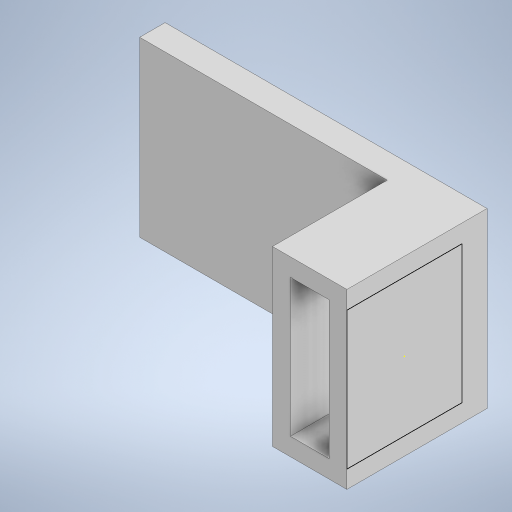
# Autodesk Inventor part: base
Saved by Autodesk Inventor 2024 (Build 280153000, 153)
## iProperties
Created: 2024-06-17
Part Number: base
Material: Generic
Document SubType Name: Modeling
Designer: omiye
Density: 1 g/cm^3
Appearance: Default
Author: omiye
Autodesk Inventor part; units mm, degrees
ref_plane "YZ Plane" through (0, 0, 0) normal (1, 0, 0) x (0, 1, 0)
ref_plane "XZ Plane" through (0, 0, 0) normal (0, 1, 0) x (-1, 0, 0)
ref_plane "XY Plane" through (0, 0, 0) normal (0, 0, 1) x (1, 0, 0)
sketch "Sketch1" plane through (0, 0, 0) normal (1, 0, 0) x (0, 1, 0)
  line L0 (27.1, -22.6) -> (-27.1, -22.6)
  line L1 (-27.1, -22.6) -> (-27.1, 22.6)
  line L2 (-27.1, 22.6) -> (27.1, 22.6)
  line L3 (27.1, 22.6) -> (27.1, -22.6)
  line L4 (27.1, -22.6) -> (-27.1, 22.6) construction
  line L5 (-27.1, -22.6) -> (27.1, 22.6) construction
  point P0 (0, 0)
  dimension "d0" = 54.2
  dimension "d1" = 45.2
  constraints: 12 end point, 2 midpoint, 2 parallel, 1 horizontal, 1 perpendicular
  measures "d0" distance of L1.end L2.end
  measures "d1" distance of L0.end L1.end
extrude "Extrusion1" add sketch "Sketch1" along normal blind 15.3
sketch "Sketch2" plane through (0, 27.1, 22.6) normal (0, 1, 0) x (1, 0, 0)
  line L0 (15.3, 0) -> (15.3, 45.2) projected
  line L1 (0, 0) -> (0, 45.2) projected
  line L2 (15.3, 0) -> (0, 0)
  line L3 (0, 0) -> (0, 45.2)
  line L4 (0, 45.2) -> (15.3, 45.2)
  line L5 (15.3, 45.2) -> (15.3, 0)
  point P0 (0, 22.6)
  constraints: 8 end point, 2 parallel, 1 horizontal, 1 perpendicular
extrude "Extrusion2" add sketch "Sketch2" along normal blind 7
sketch "Sketch3" plane through (0, -27.1, -22.6) normal (0, -1, 0) x (1, 0, 0)
  line L0 (0, 45.2) -> (0, 0) projected
  line L1 (15.3, 45.2) -> (15.3, 0) projected
  line L2 (0, 45.2) -> (15.3, 45.2)
  line L3 (15.3, 45.2) -> (15.3, 0)
  line L4 (15.3, 0) -> (0, 0)
  line L5 (0, 0) -> (0, 45.2)
  point P0 (0, 22.6)
  constraints: 8 end point, 2 parallel, 1 horizontal, 1 perpendicular
extrude "Extrusion3" add sketch "Sketch3" along normal blind 7
sketch "Sketch4" plane through (15.3, 0, 0) normal (1, 0, 0) x (0, 0, -1)
  line L0 (-22.6, -34.1) -> (-22.6, 34.1) projected
  line L1 (-22.6, 34.1) -> (22.6, 34.1) projected
  line L2 (-22.6, -34.1) -> (22.6, -34.1)
  line L3 (22.6, -34.1) -> (22.6, 34.1)
  line L4 (22.6, 34.1) -> (-22.6, 34.1)
  line L5 (-22.6, 34.1) -> (-22.6, -34.1)
  point P0 (0, 0)
  constraints: 8 end point, 2 parallel, 1 horizontal, 1 perpendicular
extrude "Extrusion4" add sketch "Sketch4" along normal blind 7
sketch "Sketch5" plane through (0, 0, 0) normal (-1, 0, 0) x (0, 0, 1)
  line L0 (-22.6, 34.1) -> (22.6, 34.1) projected
  line L1 (22.6, -34.1) -> (-22.6, -34.1) projected
  line L2 (22.6, 34.1) -> (-22.6, 34.1)
  line L3 (-22.6, 34.1) -> (-22.6, -34.1)
  line L4 (-22.6, -34.1) -> (22.6, -34.1)
  line L5 (22.6, -34.1) -> (22.6, 34.1)
  point P0 (0, 0)
  constraints: 8 end point, 2 parallel, 1 horizontal, 1 perpendicular
extrude "Extrusion5" add sketch "Sketch5" along normal blind 7
sketch "Sketch6" plane through (22.3, -34.1, -22.6) normal (0, 0, -1) x (-1, 0, 0)
  line L0 (29.3, 0) -> (0, 0) projected
  line L1 (0, 68.2) -> (0, 0) projected
  line L2 (29.3, 0) -> (0, 0)
  line L3 (0, 0) -> (0, 68.2)
  line L4 (0, 68.2) -> (29.3, 68.2)
  line L5 (29.3, 68.2) -> (29.3, 0)
  point P0 (22.3, 34.1)
  constraints: 8 end point, 2 parallel, 1 horizontal, 1 perpendicular
extrude "Extrusion6" add sketch "Sketch6" along normal blind 10
sketch "Sketch7" plane through (-7, 0, 0) normal (-1, 0, 0) x (0, 0, 1)
  line L0 (22.6, 34.1) -> (-32.6, 34.1) projected
  line L1 (22.6, -34.1) -> (-32.6, -34.1) projected
  line L2 (-32.6, 34.1) -> (-22.6, 34.1)
  line L3 (-22.6, 34.1) -> (-22.6, -34.1)
  line L4 (-22.6, -34.1) -> (-32.6, -34.1)
  line L5 (-32.6, -34.1) -> (-32.6, 34.1)
  point P0 (0, 0)
  dimension "d14" = 10
  constraints: 8 end point, 2 parallel, 1 horizontal, 1 perpendicular, 1 point on line
  measures "d14" distance of L3.end L4.end
extrude "Extrusion7" add sketch "Sketch7" along normal blind 97.5
sketch "Sketch8" plane through (22.3, -34.1, 22.6) normal (0, 0, 1) x (1, 0, 0)
  line L0 (0, 68.2) -> (-126.8, 68.2) projected
  line L1 (-29.3, 0) -> (-29.3, 68.2) projected
  line L2 (0, 68.2) -> (-29.3, 68.2)
  line L3 (-29.3, 68.2) -> (-29.3, 0)
  line L4 (-29.3, 0) -> (0, 0)
  line L5 (0, 0) -> (0, 68.2)
  line L6 (-22.25, 7) -> (-7.05, 7)
  line L7 (-7.05, 7) -> (-7.05, 61.2)
  line L8 (-7.05, 61.2) -> (-22.25, 61.2)
  line L9 (-22.25, 61.2) -> (-22.25, 7)
  line L10 (-22.25, 7) -> (-7.05, 61.2) construction
  line L11 (-7.05, 7) -> (-22.25, 61.2) construction
  point P0 (-22.3, 34.1)
  point P1 (-14.65, 34.1)
  dimension "d17" = 15.2
  dimension "d18" = 54.2
  constraints: 20 end point, 4 parallel, 2 horizontal, 2 midpoint, 2 perpendicular
  measures "d17" distance of L8.end L7.end
  measures "d18" distance of L7.end L6.end
extrude "Extrusion8" cut sketch "Sketch8" against normal blind 45.2 contours L9 L8 L7 L6
sketch "Sketch9" plane through (22.3, 0, 0) normal (1, 0, 0) x (0, 0, -1)
  line L0 (-22.6, -27.1) -> (22.6, -27.1) projected
  line L1 (-22.6, 27.1) -> (22.6, 27.1) projected
  line L2 (-22.6, -27.1) -> (22.6, -27.1)
  line L3 (22.6, -27.1) -> (22.6, 27.1)
  line L4 (22.6, 27.1) -> (-22.6, 27.1)
  line L5 (-22.6, 27.1) -> (-22.6, -27.1)
  point P0 (0, 0)
  constraints: 8 end point, 2 parallel, 1 horizontal, 1 perpendicular
body "Solid1"
